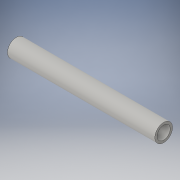
# Autodesk Inventor part: cAxelPVC1_2inchSchedule40
Saved by Autodesk Inventor 2016 SP1 (Build 200210100, 210)
## iProperties
Created: 2016-01-12
Part Number: cAxelPVC1_2inchSchedule40
Material: Generic
Document SubType Name: Modeling
Designer: steele
Density: 1 g/cm^3
Appearance: Default
Author: steele
Autodesk Inventor part; units mm, degrees
ref_plane "YZ Plane" through (0, 0, 0) normal (1, 0, 0) x (0, 1, 0)
ref_plane "XZ Plane" through (0, 0, 0) normal (0, 1, 0) x (-1, 0, 0)
ref_plane "XY Plane" through (0, 0, 0) normal (0, 0, 1) x (1, 0, 0)
sketch "Sketch3" plane through (0, 0, 0) normal (1, 0, 0) x (0, 1, 0)
  circle A0 centre (0, 0) radius 7.8994
  circle A1 centre (0, 0) radius 10.668
  dimension "d10" = 21.336
  dimension "d11" = 15.7988
  constraints: 2 centre point, 2 coincident
  measures "d10" diameter of A1
  measures "d11" diameter of A0
extrude "Extrusion3" add sketch "Sketch3" along normal blind 177.8
equation "\"d10\" = cArmOutsideDiam"
equation "\"d11\" = cArmInsideDiam"
equation "\"d12\" = cArmLength"
equation "\"cArmInsideDiam\" = 15.7988"
equation "\"cArmOutsideDiam\" = 21.336"
equation "\"cArmLength\" = 177.8"
body "Solid2"
